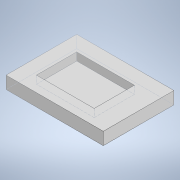
# Autodesk Inventor part: Enclosure-Bottom
Saved by Autodesk Inventor 2020 (Build 240168000, 168)
## iProperties
Created: 2019-07-15
Part Number: Enclosure-Bottom
Material: Generic
Document SubType Name: Modeling
Designer: tyrre
Density: 1 g/cm^3
Appearance: Default
Author: tyrre
Autodesk Inventor part; units mm, degrees
ref_plane "YZ Plane" through (0, 0, 0) normal (1, 0, 0) x (0, 1, 0)
ref_plane "XZ Plane" through (0, 0, 0) normal (0, 1, 0) x (-1, 0, 0)
ref_plane "XY Plane" through (0, 0, 0) normal (0, 0, 1) x (1, 0, 0)
sketch "Sketch5" plane through (0, 0, 0) normal (0, 0, 1) x (1, 0, 0)
  line L0 (-32, -5) -> (32, -5)
  line L1 (32, -5) -> (32, 5)
  line L2 (32, 5) -> (-32, 5)
  line L3 (-32, 5) -> (-32, -5)
  line L4 (-32, -5) -> (32, 5) construction
  line L5 (32, -5) -> (-32, 5) construction
  point P0 (0, 0)
  dimension "d17" = 64
  dimension "d18" = 10
  constraints: 12 end point, 2 midpoint, 2 parallel, 1 horizontal, 1 perpendicular
  measures "d17" distance of L2.end L1.end
  measures "d18" distance of L1.end L0.end
extrude "Extrusion5" add sketch "Sketch5" along normal mid plane 46.5
sketch "Sketch17" plane through (-32, 5, 23.25) normal (0, 1, 0) x (1, 0, 0)
  line L0 (0, 46.5) -> (0, 0) projected
  line L1 (0, 23.25) -> (10, 23.25)
  line L2 (10, 23.25) -> (10, 10)
  line L3 (10, 10) -> (10, 36.5)
  line L4 (10, 36.5) -> (48, 36.5)
  line L5 (48, 36.5) -> (48, 10)
  line L6 (48, 10) -> (10, 10)
  point P0 (32, 23.25)
  dimension "d84" = 10
  dimension "d85" = 13.25
  dimension "d86" = 26.5
  dimension "d87" = 38
  constraints: 12 end point, 2 parallel, 1 horizontal, 1 midpoint, 1 perpendicular, 1 point on line, 1 vertical
  measures "d84" distance of L1.start L1.end
  measures "d85" distance of L1.end L2.end
  measures "d86" distance of L2.end L3.end
  measures "d87" distance of L3.end L4.end
extrude "Extrusion15" cut sketch "Sketch17" against normal blind 5.2
sketch "Sketch18" plane through (-32, -5, 23.25) normal (-1, 0, 0) x (0, 0, 1)
  line L0 (-46.5, 0) -> (-46.5, 10) projected
  line L1 (0, 10) -> (0, 0) projected
  line L2 (-46.5, 0) -> (0, 0)
  line L3 (0, 0) -> (0, 1.8)
  line L4 (0, 1.8) -> (-46.5, 1.8)
  line L5 (-46.5, 1.8) -> (-46.5, 0)
  point P0 (-23.25, 5)
  point P1 (0, 1.8)
  point P2 (-46.5, 1.8)
  dimension "d90" = 1.8
  constraints: 8 end point, 2 parallel, 1 horizontal, 1 perpendicular
  measures "d90" distance of L3.end L1.end
extrude "Extrusion16" cut sketch "Sketch18" against normal through all
body "Solid2"
